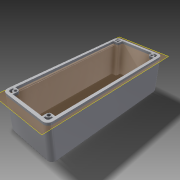
# Autodesk Inventor part: Box_Body
Saved by Autodesk Inventor 2016 (Build 200138000, 138)
## iProperties
Created: 2015-06-05
Part Number: Box_Body
Material: ABS Plastic
Document SubType Name: Modeling
Designer: Yann
Density: 1.06 g/cm^3
Appearance: Smooth - White
Author: Yann
Autodesk Inventor part; units mm, degrees
ref_plane "YZ Plane" through (0, 0, 0) normal (1, 0, 0) x (0, 1, 0)
sketch "Sketch1" plane through (0, 0, 0) normal (0, 0, 1) x (1, 0, 0)
  line L0 (0, 95.9497) -> (0, -95.9497) construction
  line L1 (-39.9497, 0) -> (39.9497, 0) construction
  arc A0 (22.5, -67.5) -> (27.5, -62.5) centre (22.5, -62.5) ccw
  line L2 (27.5, -62.5) -> (27.5, 62.5)
  arc A1 (27.5, 62.5) -> (22.5, 67.5) centre (22.5, 62.5) ccw
  line L3 (22.5, 67.5) -> (-22.5, 67.5)
  arc A2 (-22.5, 67.5) -> (-27.5, 62.5) centre (-22.5, 62.5) ccw
  line L4 (-27.5, 62.5) -> (-27.5, -62.5)
  arc A3 (-27.5, -62.5) -> (-22.5, -67.5) centre (-22.5, -62.5) ccw
  line L5 (-22.5, -67.5) -> (22.5, -67.5)
  line L6 (24.5, 62.5) -> (24.5, -62.5)
  arc A4 (22.5, -64.5) -> (24.5, -62.5) centre (22.5, -62.5) ccw
  line L7 (22.5, -64.5) -> (-22.5, -64.5)
  arc A5 (-24.5, -62.5) -> (-22.5, -64.5) centre (-22.5, -62.5) ccw
  line L8 (-24.5, -62.5) -> (-24.5, 62.5)
  arc A6 (-22.5, 64.5) -> (-24.5, 62.5) centre (-22.5, 62.5) ccw
  line L9 (-22.5, 64.5) -> (22.5, 64.5)
  arc A7 (24.5, 62.5) -> (22.5, 64.5) centre (22.5, 62.5) ccw
  circle A8 centre (20.5, 60.5) radius 2.5 construction
  line L10 (20.5, 58) -> (24.5, 58)
  line L11 (18, 60.5) -> (18, 64.5)
  line L12 (22.9495, 60) -> (24.5, 60)
  line L13 (20, 62.9495) -> (20, 64.5)
  circle A9 centre (20.5, 60.5) radius 1.5
  arc A10 (22.9495, 60) -> (20, 62.9495) centre (20.5, 60.5) ccw
  arc A11 (18, 60.5) -> (20.5, 58) centre (20.5, 60.5) ccw
  circle A12 centre (20.5, -60.5) radius 2.5 construction
  line L14 (20.5, -58) -> (24.5, -58)
  line L15 (18, -60.5) -> (18, -64.5)
  line L16 (22.9495, -60) -> (24.5, -60)
  line L17 (20, -62.9495) -> (20, -64.5)
  circle A13 centre (20.5, -60.5) radius 1.5
  arc A14 (20, -62.9495) -> (22.9495, -60) centre (20.5, -60.5) ccw
  arc A15 (20.5, -58) -> (18, -60.5) centre (20.5, -60.5) ccw
  circle A16 centre (-20.5, 60.5) radius 2.5 construction
  line L18 (-20.5, 58) -> (-24.5, 58)
  line L19 (-18, 60.5) -> (-18, 64.5)
  line L20 (-22.9495, 60) -> (-24.5, 60)
  line L21 (-20, 62.9495) -> (-20, 64.5)
  circle A17 centre (-20.5, 60.5) radius 1.5
  arc A18 (-20, 62.9495) -> (-22.9495, 60) centre (-20.5, 60.5) ccw
  arc A19 (-20.5, 58) -> (-18, 60.5) centre (-20.5, 60.5) ccw
  line L22 (-20.5, -58) -> (-24.5, -58)
  arc A20 (-18, -60.5) -> (-20.5, -58) centre (-20.5, -60.5) ccw
  line L23 (-22.9495, -60) -> (-24.5, -60)
  circle A21 centre (-20.5, -60.5) radius 1.5
  line L24 (-18, -60.5) -> (-18, -64.5)
  circle A22 centre (-20.5, -60.5) radius 2.5 construction
  arc A23 (-22.9495, -60) -> (-20, -62.9495) centre (-20.5, -60.5) ccw
  line L25 (-20, -62.9495) -> (-20, -64.5)
  line L26 (-24.5, 60) -> (-24.5, 58)
  line L27 (-20, 64.5) -> (-18, 64.5)
  line L28 (24.5, -58) -> (24.5, -60)
  line L29 (18, -64.5) -> (20, -64.5)
  line L30 (-20, -64.5) -> (-18, -64.5)
  line L31 (-24.5, -58) -> (-24.5, -60)
  point P0 (-22.5, -62.5)
  point P1 (-22.5, 62.5)
  dimension "d6" = 3
  dimension "d7" = 5
  dimension "d8" = 7
  dimension "d9" = 7
  dimension "d10" = 2
  dimension "d11" = 2
  dimension "d12" = 3
  dimension "d20" = 55
  dimension "d21" = 135
  dimension "d22" = 5
  constraints: 60 end point, 48 point on circle, 38 symmetric about line, 24 centre point, 12 coincident, 10 tangent, 6 collinear, 5 point on line, 4 perpendicular, 2 equal radius, 20 other
  measures "d6" distance between parallel lines of L6 L2
  measures "d7" diameter of A8
  measures "d8" distance from line of L2 A8.centre
  measures "d9" distance from line of L3 A8.centre
  measures "d10" distance between parallel lines of L10 L12
  measures "d11" distance between parallel lines of L13 L11
  measures "d12" diameter of A9
  measures "d20" distance between parallel lines of L4 L2
  measures "d21" distance between parallel lines of L5 L3
  measures "d22" radius of A1
ref_plane "Work Plane4" through (-27.5, -67.5, 0) normal (0, 0, -1) x (0, 1, 0)
ref_plane "Work Plane5" through (-27.5, -67.5, -58.6068) normal (0, 0, 1) x (1, 0, 0)
extrude "Extrusion1" add sketch "Sketch1" against normal blind 38.75 contours L5 A3 L4 A2 L3 A1 L2 A0 | L6 L10 A11 L11 L9 L13 A10 L12 | L6 L16 A14 L17 L7 L15 A15 L14 | L19 A19 L18 L8 L20 A18 L21 L9 | L7 L25 A23 L23 L8 L22 A20 L24
ref_plane "PLan support PowerPCB" through (0, 0, -2.7) normal (0, 0, 1) x (1, 0, 0)
sketch "Sketch2" plane through (0, 0, -2.7) normal (0, 0, 1) x (1, 0, 0)
  line L0 (24.5, 58) -> (24.5, -58) projected
  line L1 (22.5, 58) -> (22.5, -58)
  line L2 (24.5, 58) -> (22.5, 58)
  line L3 (24.5, -58) -> (22.5, -58)
  line L4 (0, 94.5) -> (0, -94.5) construction
  line L5 (-24.5, 58) -> (-24.5, -58)
  line L6 (-22.5, 58) -> (-22.5, -58)
  line L7 (-24.5, 58) -> (-22.5, 58)
  line L8 (-24.5, -58) -> (-22.5, -58)
  point P0 (0, 0)
  dimension "d15" = 2
  constraints: 16 end point, 4 symmetric about line, 2 perpendicular, 1 parallel, 1 vertical, 2 other
  measures "d15" distance between parallel lines of L0 L1
extrude "Extrusion2" add sketch "Sketch2" against normal blind 2.5
fillet "Fillet1" radius 2 2 edges at (-22.5, 0, -5.2) (22.5, 0, -5.2)
equation "\"d9\" = d8"
equation "\"d11\" = d10"
equation "\"d13\" = -Top_Plate_Bottom_to_PowerPcb_Bottom"
equation "\"Plate_thickness\" = 3"
equation "\"Top_Plate_Bottom_to_PowerPcb_Bottom\" = 2.7"
body "Solid1"
